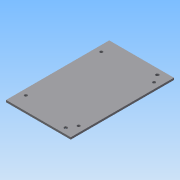
# Autodesk Inventor part: redboard_plate
Saved by Autodesk Inventor 2015 (Build 190159000, 159)
## iProperties
Created: 2014-12-13
Part Number: redboard_plate
Material: Generic
Document SubType Name: Modeling
Designer: Daniel
Density: 1 g/cm^3
Appearance: Default
Author: Daniel
Autodesk Inventor part; units mm, degrees
ref_plane "YZ Plane" through (0, 0, 0) normal (1, 0, 0) x (0, 1, 0)
ref_plane "XZ Plane" through (0, 0, 0) normal (0, 1, 0) x (-1, 0, 0)
ref_plane "XY Plane" through (0, 0, 0) normal (0, 0, 1) x (1, 0, 0)
sketch "Sketch1" plane through (0, 0, 0) normal (0, 1, 0) x (-1, 0, 0)
  line L0 (0, 0) -> (76.2, 0)
  line L1 (76.2, 0) -> (76.2, -121.539)
  line L2 (76.2, -121.539) -> (0, -121.539)
  line L3 (0, -121.539) -> (0, 0)
  dimension "d0" = 76.2
  dimension "d1" = 121.539
  constraints: 8 end point, 2 parallel, 1 horizontal, 1 perpendicular
  measures "d0" distance of L1.end L2.end
  measures "d1" distance of L0.end L1.end
extrude "Extrusion1" add sketch "Sketch1" along normal blind 2.3813
sketch "Sketch2" plane through (0, 2.3813, 0) normal (0, 1, 0) x (1, 0, 0)
  line L0 (-6.985, -6.7053) -> (-6.985, 140.88) construction
  line L1 (-69.215, -6.7053) -> (-69.215, 134.4303) construction
  line L2 (-84.4429, 16.3195) -> (15.1684, 16.3195) construction
  line L3 (-82.9542, 105.2195) -> (32.716, 105.2195) construction
  line L4 (-85.3039, 60.7695) -> (24.2122, 60.7695) construction
  line L5 (-38.1, -11.6346) -> (-38.1, 148.7845) construction
  line L6 (-76.2, 121.539) -> (-76.2, 0) construction
  line L7 (-76.2, 0) -> (0, 0) construction
  point P0 (-76.2, 60.7695)
  point P1 (-38.1, 0)
  point P2 (-69.215, 16.3195)
  point P3 (-6.985, 16.3195)
  point P4 (-6.985, 105.2195)
  point P5 (-69.215, 105.2195)
  dimension "d4" = 88.9
  dimension "d5" = 62.23
  constraints: 12 end point, 10 point on line, 3 horizontal, 3 vertical, 2 midpoint, 2 other
  measures "d4" diameter of L2 L4
  measures "d5" diameter of L1 L5
hole "Hole1" at (-69.215, 2.3813, -16.3195) at (-6.985, 2.3813, -16.3195) at (-6.985, 2.3813, -105.2195) at (-69.215, 2.3813, -105.2195) direction (0, -1, 0) diameter 3.4544 depth 25.4 tip angle 118 clearance for "Flat Head Machine Screw (82)" size "#5" standard "Ansi Unified Screw Threads"
sketch "Sketch3" plane through (0, 2.3813, 0) normal (0, 1, 0) x (1, 0, 0)
  line L0 (-12.7, -7.2404) -> (-12.7, 131.1471) construction
  line L1 (0, 0) -> (0, 121.539) construction
  line L2 (-88.3446, 60.7695) -> (40.5312, 60.7695) construction
  point P0 (-12.7, 6.7945)
  point P1 (-12.7, 114.7445)
  point P2 (0, 60.7695)
  dimension "d13" = 12.7
  dimension "d14" = 107.95
  constraints: 4 end point, 3 point on line, 1 horizontal, 1 midpoint, 1 symmetric about line, 1 vertical
  measures "d13" distance between parallel lines of L0 L1
  measures "d14" diameter of point (-12.7, 6.795) L2
hole "Hole2" at (-12.7, 2.3813, -6.7945) at (-12.7, 2.3813, -114.7445) direction (0, -1, 0) diameter 3.81 depth 25.4 tip angle 118 clearance for "Flat Head Machine Screw (82)" size "#6" standard "Ansi Unified Screw Threads"
body "Solid1"
